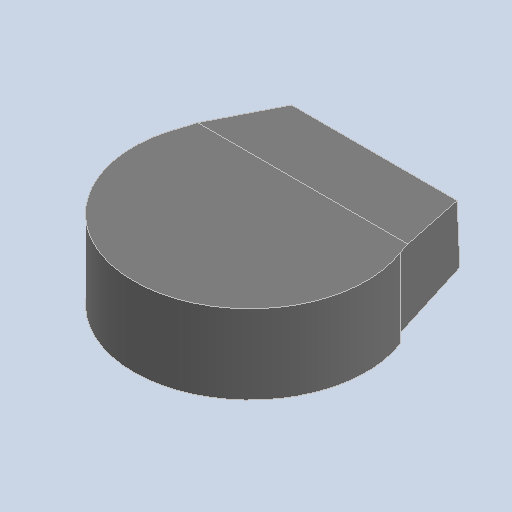
# Autodesk Inventor part: vez
Saved by Autodesk Inventor 2022 (Build 260153000, 153)
## iProperties
Created: 2022-11-29
Part Number: vez
Material: Generic
Document SubType Name: Modeling
Designer: matys
Density: 1 g/cm^3
Appearance: Gray
Author: matys
Autodesk Inventor part; units mm, degrees
ref_plane "YZ Plane" through (0, 0, 0) normal (1, 0, 0) x (0, 1, 0)
ref_plane "XZ Plane" through (0, 0, 0) normal (0, 1, 0) x (-1, 0, 0)
ref_plane "XY Plane" through (0, 0, 0) normal (0, 0, 1) x (1, 0, 0)
sketch "Sketch1" plane through (0, 0, 0) normal (0, 1, 0) x (-1, 0, 0)
  arc A0 (46.7415, -17.825) -> (-46.7415, -17.825) centre (0, 0) ccw
  line L0 (0, 0) -> (0, -55.2)
  line L1 (0, -55.2) -> (35.075, -55.2)
  line L2 (0, -55.2) -> (-35.075, -55.2)
  line L3 (0, 50.025) -> (0, -17.825)
  line L4 (0, -17.825) -> (46.7415, -17.825)
  line L5 (35.075, -55.2) -> (46.7415, -17.825)
  line L6 (0, -17.825) -> (-46.7415, -17.825)
  line L7 (-35.075, -55.2) -> (-46.7415, -17.825)
  line L8 (50.025, 0) -> (48.025, 0)
  arc A1 (44.5945, -17.825) -> (-44.5945, -17.825) centre (0, 0) ccw
  line L9 (35.075, -55.2) -> (33.075, -55.2)
  line L10 (33.075, -55.2) -> (44.5945, -17.825)
  line L11 (-35.075, -55.2) -> (-46.7415, -17.825)
  line L12 (-33.075, -55.2) -> (-44.5945, -17.825)
  dimension "d0" = 100.05
  dimension "d1" = 55.2
  dimension "d2" = 35.075
  dimension "d3" = 35.075
  dimension "d4" = 67.85
  dimension "d5" = 2
  dimension "d6" = 2
  constraints: 26 end point, 7 point on circle, 4 point on line, 3 horizontal, 2 centre point, 2 coincident, 2 symmetric about line, 1 perpendicular, 1 vertical
  measures "d0" diameter of A0
  measures "d1" distance of L0.start L0.end
  measures "d2" distance of L0.end L1.end
  measures "d3" distance of L0.end L2.end
  measures "d4" distance of L3.start L3.end
  measures "d5" distance of L8.start L8.end
  measures "d6" distance of L1.end L9.end
extrude "Extrusion1" add sketch "Sketch1" along normal blind 30
chamfer "Chamfer1" distance 2 distance2 30 2 edges at (-17.5375, 30, -55.2) (17.5375, 30, -55.2)
chamfer "Chamfer2" distance 4 distance2 30.5 2 edges at (-17.8496, 30, -53.2) (17.8496, 30, -53.2)
sketch "Sketch2" plane through (0, 0, 0) normal (0, -1, 0) x (1, 0, 0)
  arc A0 (46.7415, -17.825) -> (-46.7415, -17.825) centre (0, 0) ccw projected
  line L0 (28.4099, 41.175) -> (28.4099, 39.175)
  line L1 (28.4099, 41.175) -> (28.4099, -17.825)
  line L2 (-46.7415, -22.7) -> (46.7415, -22.7) projected
  line L3 (28.4099, -17.825) -> (46.7415, -17.825)
  line L4 (46.7415, -17.825) -> (-46.7415, -17.825)
  arc A1 (46.7415, -17.825) -> (-46.7415, -17.825) centre (0, 0) ccw
  line L5 (0, 0) -> (28.4099, 9.6374)
  circle A2 centre (0, 0) radius 30
  circle A3 centre (0, 0) radius 36.8
  line L6 (0, -36.8) -> (0, -40.8)
  line L7 (35.075, -55.2) -> (-35.075, -55.2) projected
  line L8 (4.575, -55.2) -> (35.075, -55.2)
  line L9 (35.075, -55.2) -> (19.825, -55.2)
  line L10 (-15.25, -40.8) -> (-46.7415, -17.825)
  line L11 (-15.25, -40.8) -> (0, -40.8)
  circle A4 centre (0, 0) radius 37.375
  line L12 (15.25, -40.8) -> (46.7415, -17.825)
  line L13 (15.25, -40.8) -> (0, -40.8)
  point P0 (-46.7415, -17.825)
  point P1 (28.4099, -9.6374)
  point P2 (24.1303, -17.825)
  point P3 (-24.1303, -17.825)
  point P4 (46.7415, -17.825)
  dimension "d18" = 73.6
  dimension "d15" = 2
  dimension "d16" = 59
  dimension "d17" = 30
  dimension "d19" = 4
  dimension "d24" = 74.75
  constraints: 24 end point, 3 coincident, 3 point on circle, 3 vertical, 2 centre point, 2 symmetric about line, 1 collinear, 1 midpoint, 1 parallel, 1 perpendicular, 1 point on line, 1 vertical alignment, 6 other
  measures "d15" distance of L0.start L0.end
  measures "d16" distance of L0.start L1.end
  measures "d17" distance of L5.start L5.end
  measures "d19" distance of L6.start L6.end
  measures "d24" diameter of A4
extrude "Extrusion2" add sketch "Sketch2" along normal blind 4 contours L3 A4 L1 L0 A0 | L12 L2 A4 L3 | L0 L1 A4 L4 A0 | L12 L13 L6 A4 L2 | L4 A4 L2 L10 | L2 A4 L6 L11 L10
sketch "Sketch3" plane through (0, -4, 0) normal (0, -1, 0) x (1, 0, 0)
  line L0 (0, 0) -> (0, 30)
  circle A0 centre (0, 0) radius 30
  line L1 (0, 30) -> (0, 32.5)
  circle A1 centre (0, 0) radius 32.5
  dimension "d22" = 30
  dimension "d25" = 2.5
  constraints: 4 end point, 2 coincident, 2 point on circle, 2 vertical, 1 centre point, 1 vertical alignment, 2 other
  measures "d22" distance of L0.start L0.end
  measures "d25" distance of L1.start L1.end
extrude "Extrusion3" add sketch "Sketch3" along normal blind 5
sketch "Sketch4" plane through (0, -9, 0) normal (0, -1, 0) x (1, 0, 0)
  circle A0 centre (0, 0) radius 32.5 projected
  line L0 (0, 32.5) -> (0, 37.5)
  circle A1 centre (0, 0) radius 37.5
  arc A2 (28.4099, -9.6374) -> (28.4099, 9.6374) centre (0, 0) ccw projected
  line L1 (0, 30) -> (0, 26.5)
  circle A3 centre (0, 0) radius 26.5
  point P0 (-24.1303, -17.825)
  point P1 (24.1303, -17.825)
  dimension "d28" = 5
  dimension "d29" = 3.5
  constraints: 4 end point, 3 vertical alignment, 2 coincident, 2 vertical, 1 point on circle, 5 other
  measures "d28" distance of L0.start L0.end
  measures "d29" distance of L1.start L1.end
extrude "Extrusion4" add sketch "Sketch4" along normal blind 5 contours A0 | A1
sketch "Sketch5" plane through (0, -4, 0) normal (0, -1, 0) x (1, 0, 0)
  arc A0 (9.6374, 28.4099) -> (-9.6374, 28.4099) centre (0, 0) ccw projected
  line L0 (0, 30) -> (0, 26.5)
  circle A1 centre (0, 0) radius 26.5 projected
  circle A2 centre (0, 0) radius 30
  circle A3 centre (0, 0) radius 32.5
  point P0 (-24.1303, -17.825)
  point P1 (24.1303, -17.825)
  constraints: 2 centre point, 2 coincident, 2 end point, 1 concentric, 1 point on circle, 1 vertical, 1 vertical alignment, 1 other
extrude "Extrusion5" cut sketch "Sketch5" against normal blind 30 contours A1
sketch "Sketch6" plane through (0, -14, 0) normal (0, -1, 0) x (1, 0, 0)
  circle A0 centre (0, 0) radius 37.5
  constraints: 1 centre point, 1 coincident
extrude "Extrusion6" cut sketch "Sketch6" against normal blind 10
sketch "Sketch7" plane through (0, -4, 0) normal (0, -1, 0) x (1, 0, 0)
  circle A0 centre (0, 0) radius 30
  circle A1 centre (0, 0) radius 30 projected
  line L0 (0, -30) -> (0, -32.5)
  line L1 (41.0682, -36) -> (-15.25, -36) projected
  circle A2 centre (0, 0) radius 32.5
  line L2 (30, 0) -> (33.5, 0)
  circle A3 centre (0, 0) radius 33.5
  point P0 (15.25, -36)
  dimension "d36" = 2.5
  dimension "d44" = 3.5
  constraints: 4 end point, 3 coincident, 2 point on circle, 1 centre point, 1 horizontal, 1 horizontal alignment, 1 perpendicular, 1 vertical alignment, 4 other
  measures "d36" distance of L0.start L0.end
  measures "d44" distance of L2.start L2.end
extrude "Extrusion7" cut sketch "Sketch7" against normal blind 5 contours L2 A2 L0 A0 | A0 L0 A2 L2 | A3
sketch "Sketch8" plane through (0, 1, 0) normal (0, -1, 0) x (1, 0, 0)
  circle A0 centre (0, 0) radius 30
  line L0 (32.5, 0) -> (-32.5, 0)
  line L1 (33.3654, -3) -> (-33.3654, -3)
  line L2 (33.3654, 3) -> (-33.3654, 3)
  line L3 (30, 0) -> (33.5, 0)
  circle A1 centre (0, 0) radius 33.5
  circle A2 centre (0, 0) radius 33.5 projected
  circle A3 centre (0, 0) radius 33.5
  point P0 (-29.8496, -3)
  point P1 (-29.8496, 3)
  point P2 (29.8496, 3)
  point P3 (29.8496, -3)
  dimension "d39" = 3
  dimension "d40" = 3
  dimension "d43" = 3.5
  constraints: 8 end point, 4 point on circle, 3 coincident, 2 horizontal, 2 parallel, 1 centre point, 1 horizontal alignment, 1 point on line, 6 other
  measures "d39" distance between parallel lines of L0 L1
  measures "d40" distance between parallel lines of L0 L2
  measures "d43" distance of L3.start L3.end
extrude "Extrusion8" cut sketch "Sketch8" against normal blind 5 contours L0 L3 A1 L1 A0 | A0 L2 A1 L3 L0 | A0 L1 A1 L2
sketch "Sketch9" plane through (0, -4, 0) normal (0, -1, 0) x (1, 0, 0)
  point P0 (0, 0)
ref_plane "Work Plane1" through (-46.7415, 15, -17.825) normal (0, 0, -1) x (-1, 0, 0)
sketch "Sketch12" plane through (-46.7415, 15, -17.825) normal (0, 0, -1) x (-1, 0, 0)
  line L0 (-82.3578, 11.0089) -> (-81.8165, -15) projected
  line L1 (-11.6665, -15) -> (-11.1253, 11.0089) projected
  line L2 (-81.8165, -15) -> (-11.6665, -15)
  line L3 (-11.6665, -15) -> (-11.6665, 11.0089)
  line L4 (-82.3578, 11.0089) -> (-11.1253, 11.0089) projected
  line L5 (-93.483, -15) -> (-81.8165, -15) projected
  line L6 (-81.8165, -15) -> (-81.8165, 11.0089)
  line L7 (-81.8165, -15) -> (-81.8165, 11.0089)
  line L8 (-81.8165, 11.0089) -> (-16.7415, 11.0089)
  line L9 (-16.7415, -9) -> (-16.7415, 11) projected
  line L10 (-81.8165, -15) -> (-11.6665, -15) projected
  line L11 (-81.8165, -15) -> (-78.8165, -15)
  line L12 (-78.8165, -15) -> (-78.8165, -12)
  line L13 (-78.8165, -12) -> (-81.8165, -12)
  line L14 (-11.6665, -15) -> (-11.6665, 11.0089)
  line L15 (-11.6665, 11.0089) -> (-11.6665, 8.0089)
  line L16 (-11.6665, 8.0089) -> (-14.6665, 8.0089)
  line L17 (-14.6665, 8.0089) -> (-78.8165, 8.0089)
  line L18 (-78.8165, 8.0089) -> (-78.8165, -12)
  line L19 (-78.8165, -12) -> (-14.6665, -12)
  line L20 (-14.6665, -12) -> (-14.6665, 8.0089)
  point P0 (-46.7415, -15)
  dimension "d47" = 3
  dimension "d48" = 3
  dimension "d49" = 3
  dimension "d50" = 3
  constraints: 30 end point, 7 point on line, 6 perpendicular, 4 equal length, 2 horizontal
  measures "d47" distance of L0.end L11.end
  measures "d48" distance of L11.end L12.end
  measures "d49" distance of L3.end L15.end
  measures "d50" distance of L15.end L16.end
extrude "Extrusion9" [suppressed]
sketch "Sketch13" plane through (32.075, 3, -11.9896) normal (-1, 0, 0) x (0, 0, 1)
  line L0 (-43.0104, 0) -> (-41.6765, 20.0089) projected
  line L1 (-43.0104, 0) -> (-41.6765, 20.0089)
  line L2 (-43.0104, 0) -> (-42.3435, 10.0044)
  line L3 (-42.3435, 10.0044) -> (-5.8354, 10.0044)
  line L4 (-5.8354, -3) -> (-5.8354, 27) projected
  line L5 (-42.3435, 10.0044) -> (-37.3435, 10.0044)
  line L6 (-37.3435, 10.0044) -> (-37.3435, 5.0044)
  line L7 (-37.3435, 5.0044) -> (-42.6769, 5.0022)
  line L8 (-37.3435, 10.0044) -> (-37.3435, 15.0044)
  line L9 (-37.3435, 15.0044) -> (-42.0101, 15.0044)
  line L10 (-37.3435, 10.0044) -> (-32.3435, 10.0044)
  line L11 (-37.3435, 10.0044) -> (-32.3435, 10.0044)
  line L12 (-32.3435, 10.0044) -> (-32.3435, 5.5044)
  circle A0 centre (-32.3435, 10.0044) radius 4.5
  point P0 (11.9896, -3)
  dimension "d55" = 5
  dimension "d56" = 5
  dimension "d57" = 5
  dimension "d58" = 5
  dimension "d59" = 4.5
  constraints: 22 end point, 5 point on line, 3 perpendicular, 2 collinear, 2 midpoint, 1 coincident, 1 horizontal, 1 vertical alignment, 2 other
  measures "d55" distance of L2.end L5.end
  measures "d56" distance of L5.end L6.end
  measures "d57" distance of L5.end L8.end
  measures "d58" distance of L5.end L10.end
  measures "d59" distance of L10.end L12.end
extrude "Extrusion10" [suppressed]
body "Solid1"
